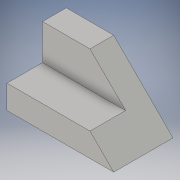
# Autodesk Inventor part: Figure 7_28_6
Saved by Autodesk Inventor 2016 (Build 200138000, 138)
## iProperties
Created: 2016-07-19
Part Number: Figure 7_28_6
Material: Generic
Document SubType Name: Modeling
Designer: cfkguest
Density: 1 g/cm^3
Appearance: Default
Author: cfkguest
Autodesk Inventor part; units mm, degrees
ref_plane "YZ Plane" through (0, 0, 0) normal (1, 0, 0) x (0, 1, 0)
ref_plane "XZ Plane" through (0, 0, 0) normal (0, 1, 0) x (-1, 0, 0)
ref_plane "XY Plane" through (0, 0, 0) normal (0, 0, 1) x (1, 0, 0)
sketch "Sketch1" plane through (0, 0, 0) normal (0, 0, 1) x (1, 0, 0)
  line L0 (-22.0262, 11.1206) -> (35.1238, 11.1206)
  line L1 (35.1238, 11.1206) -> (35.1238, -20.6294)
  line L2 (35.1238, -20.6294) -> (-22.0262, -20.6294)
  line L3 (-22.0262, -20.6294) -> (-22.0262, 11.1206)
  point P0 (0, 0)
  dimension "d0" = 57.15
  dimension "d1" = 31.75
  constraints: 8 end point, 2 parallel, 1 horizontal, 1 perpendicular
  measures "d0" distance of L0.start L0.end
  measures "d1" distance of L2.end L0.start
extrude "Extrusion1" add sketch "Sketch1" along normal blind 31.75
sketch "Sketch2" plane through (0, 0, 31.75) normal (0, 0, 1) x (1, 0, 0)
  line L0 (35.1238, 11.1206) -> (-22.0262, 11.1206) projected
  line L1 (-22.0262, 11.1206) -> (35.1238, 11.1206)
  line L2 (35.1238, 11.1206) -> (35.1238, -7.9294)
  line L3 (35.1238, -7.9294) -> (-22.0262, -7.9294)
  line L4 (-22.0262, -7.9294) -> (-22.0262, 11.1206)
  point P0 (0, 0)
  dimension "d4" = 19.05
  dimension "d5" = 57.15
  constraints: 8 end point, 2 parallel, 1 horizontal, 1 perpendicular
  measures "d4" distance of L1.end L2.end
  measures "d5" distance of L2.end L3.end
extrude "Extrusion2" cut sketch "Sketch2" against normal blind 19.05
sketch "Sketch3" plane through (0, 0, 31.75) normal (0, 0, 1) x (1, 0, 0)
  line L0 (-22.0262, -20.6294) -> (35.1238, -20.6294) projected
  line L1 (35.1238, -20.6294) -> (22.4238, -7.9294)
  line L2 (35.1238, -7.9294) -> (-22.0262, -7.9294) projected
  line L3 (22.4238, -7.9294) -> (35.1238, -7.9294)
  line L4 (35.1238, 11.1206) -> (35.1238, -20.6294) projected
  line L5 (35.1238, -7.9294) -> (35.1238, -20.6294)
  point P0 (0, 0)
  dimension "d8" = 44.45
  constraints: 6 end point, 1 collinear, 1 perpendicular, 1 point on line
  measures "d8" distance of L2.end L1.end
extrude "Extrusion3" cut sketch "Sketch3" against normal blind 19.05
sketch "Sketch4" plane through (0, 0, 0) normal (0, 0, -1) x (-1, 0, 0)
  line L0 (-35.1238, -20.6294) -> (-22.4238, -7.9294) projected
  line L1 (-35.1238, -20.6294) -> (-3.3738, 11.1206)
  line L2 (22.0262, 11.1206) -> (-35.1238, 11.1206) projected
  line L3 (-3.3738, 11.1206) -> (-35.1238, 11.1206)
  line L4 (-35.1238, 11.1206) -> (-35.1238, -20.6294) projected
  line L5 (-35.1238, 11.1206) -> (-35.1238, -20.6294)
  point P0 (0, 0)
  dimension "d11" = 25.4
  constraints: 6 end point, 2 collinear, 1 point on line
  measures "d11" distance of L2.start L1.end
extrude "Extrusion4" cut sketch "Sketch4" against normal blind 19.05
body "Solid1"
